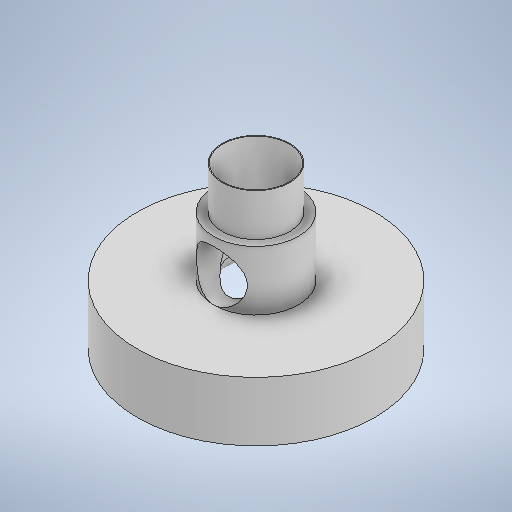
# Autodesk Inventor part: vial_adapter_male
Saved by Autodesk Inventor 2025 (Build 290162010, 162A)
## iProperties
Created: 2023-04-28
Part Number: vial_adapter_male
Material: Generic
Document SubType Name: Modeling
Designer: dinesh
Density: 1 g/cm^3
Appearance: Default
Author: dinesh
Autodesk Inventor part; units mm, degrees
ref_plane "YZ Plane" through (0, 0, 0) normal (1, 0, 0) x (0, 1, 0)
ref_plane "XZ Plane" through (0, 0, 0) normal (0, 1, 0) x (-1, 0, 0)
ref_plane "XY Plane" through (0, 0, 0) normal (0, 0, 1) x (1, 0, 0)
sketch "Sketch1" plane through (0, 0, 0) normal (0, 0, 1) x (1, 0, 0)
  line L0 (4, 8) -> (5, 8)
  line L1 (5, 8) -> (5, 1)
  line L2 (8.5, 0) -> (3, 0)
  line L3 (3, 2) -> (3, 8)
  line L4 (0, 50) -> (0, -50)
  line L5 (3, 8) -> (4, 8) construction
  line L6 (4, 8) -> (4, 13)
  line L7 (5, 1) -> (14, 1)
  line L8 (14, 1) -> (14, 0)
  line L9 (13, 0) -> (5, 0)
  line L10 (5, 0) -> (5, 1) construction
  line L11 (14, 0) -> (13, 0) construction
  line L12 (13, 0) -> (13, -6)
  line L13 (13, -6) -> (14, -6)
  line L14 (14, -6) -> (14, 0)
  line L15 (11.5, 0) -> (10.5, 0)
  arc A0 (3, 2) -> (5, 0) centre (5, 2) ccw
  line L16 (-4.4, 0) -> (4.4, 0) construction
  line L17 (10.4, 0) -> (11.4, 0)
  line L18 (11.4, 0) -> (11.4, -6)
  line L19 (11.4, -6) -> (10.4, -6) construction
  line L20 (10.4, -6) -> (10.4, -6)
  arc A1 (10.4, -6) -> (4.4, 0) centre (4.4, -6) ccw
  line L21 (4, 13) -> (3.9, 13)
  line L22 (3.9, 13) -> (3, 8)
  line L23 (11.4, -6) -> (11.4, -12)
  line L24 (11.4, -12) -> (11.3, -12)
  line L25 (11.3, -12) -> (10.4, -6)
  point P0 (0, 0)
  point P1 (11.4, 0)
  point P2 (5, 0)
  point P3 (4.4, 0)
  dimension "d0" = 6
  dimension "d1" = 8
  dimension "d2" = 10
  dimension "d5" = 1
  dimension "d6" = 26
  dimension "d7" = 1
  dimension "d8" = 6
  dimension "d11" = 2
  dimension "d12" = 100
  dimension "d15" = 1
  dimension "d16" = 1.6
  dimension "d17" = 6
  dimension "d26" = 0.1
  dimension "d27" = 1
  dimension "d28" = 5
  dimension "d29" = 6
  dimension "d30" = 0.1
  constraints: 52 end point, 8 horizontal, 8 parallel, 6 perpendicular, 4 point on circle, 4 point on line, 4 tangent, 3 collinear, 3 midpoint, 2 centre point, 2 vertical
  measures "d0" diameter of L3 L4
  measures "d1" distance between parallel lines of L0 L2
  measures "d2" diameter of L1 L4
  measures "d5" distance between parallel lines of L9 L7
  measures "d6" diameter of L12 L4
  measures "d7" distance between parallel lines of L12 L14
  measures "d8" distance between parallel lines of L13 L9
  measures "d11" radius of A0
  measures "d12" distance of L4.start L4.end
  measures "d15" distance between parallel lines of L18 L20
  measures "d16" distance between parallel lines of L12 L18
  measures "d17" radius of A1
  measures "d26" distance of L6.end L21.end
  measures "d27" distance between parallel lines of L3 L6
  measures "d28" distance of L0.start L6.end
  measures "d29" distance of L18.end L23.end
  measures "d30" distance of L23.end L24.end
revolve "Revolution1" add sketch "Sketch1" angle 360 about axis through (0, 50, 0) along (0, -1, 0) contours L0 L1 L7 L8 L14 L13 L12 L9 L2 A0 L3 L22 L21 L6
sketch "Sketch2" plane through (0, 0, 0) normal (0, 0, 1) x (1, 0, 0)
  line L0 (-2, 11) -> (2, 11) projected
  line L1 (-3, 2) -> (3, 2) construction
  line L2 (-4, 13) -> (4, 13) projected
  line L3 (0, 13) -> (0, 2) construction
  line L4 (-4, 8) -> (4, 8) projected
  circle A0 centre (0, 4) radius 3
  line L5 (-5, 0) -> (5, 0) projected
  point P0 (0, 0)
  point P1 (4, 13)
  point P2 (2.2361, 2)
  point P3 (-2.2361, 2)
  dimension "d0" = 6
  dimension "d19" = 6
  dimension "d25" = 4
  constraints: 2 end point, 1 centre point, 1 midpoint, 1 point on line, 2 other
  measures "d19" diameter of A0
  measures "d25" distance from line of L5 A0.centre
extrude "Extrusion1" cut sketch "Sketch2" along normal blind 10 and the other way blind 3.1
equation "\"d0\" = t_D"
equation "\"d1\" = top_th + w_th"
equation "\"d2\" = top_D"
equation "\"d5\" = w_th"
equation "\"d6\" = lv_OD"
equation "\"d7\" = w_th"
equation "\"d8\" = w_l"
equation "\"d11\" = fillet_D"
equation "\"d15\" = w_th"
equation "\"d16\" = lv_th"
equation "\"d17\" = 3 * fillet_D"
equation "\"d26\" = tol"
equation "\"d27\" = w_th"
equation "\"d28\" = cn_h"
equation "\"d29\" = w_l"
equation "\"d30\" = tol"
equation "\"d19\" = t_D"
equation "\"d25\" = 0.5 * t_D + w_th"
equation "\"d21\" = top_D"
equation "\"d22\" = 0.5 * t_D + tol"
equation "\"tol\" = 0.1"
equation "\"fillet_D\" = 2"
equation "\"w_th\" = 1"
equation "\"w_l\" = 6"
equation "\"t_D\" = 6"
equation "\"top_D\" = 10"
equation "\"top_th\" = t_D + w_th"
equation "\"cn_h\" = 5"
equation "\"lv_OD\" = 26"
equation "\"lv_th\" = 1.6"
equation "\"t_D_f\" = t_D + w_th"
equation "\"top_th_f\" = t_D_f + cn_h"
equation "\"sv_OD\" = 13"
equation "\"sv_th\" = 1.5"
equation "\"b_OD\" = 44"
equation "\"b_th\" = 1.5"
equation "\"b_ID\" = 36.5"
equation "\"b_rim_h\" = 5"
equation "\"h_D\" = 0.9"
equation "\"h_s\" = 2.25"
equation "\"v_h_D\" = 7.5"
equation "\"v_h_off\" = 0.5 * cn_D + 0.5 * v_h_D"
equation "\"cn_D\" = 13.2"
body "Solid1"
